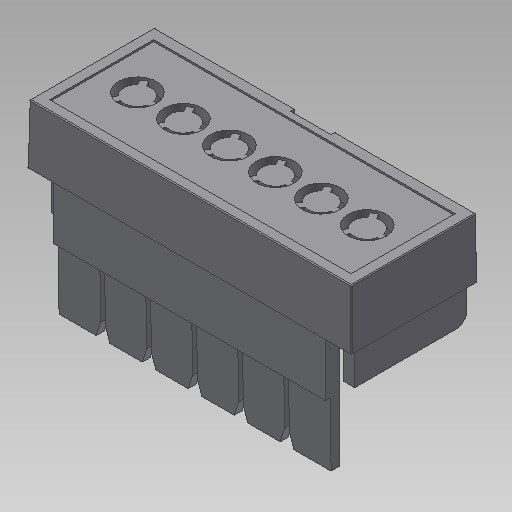
# Autodesk Inventor part: D2MG guard
Saved by Autodesk Inventor 2018 (Build 220112000, 112)
## iProperties
Created: 2015-02-09
Part Number: D2MG guard
Material: Типовые
Document SubType Name: Modeling
Designer: Abbath
Density: 1 g/cm^3
Appearance: По умолчанию
Mass: 2.0666 g
Surface Area: 34.2818 cm^2
Volume: 2.0666 cm^3
Author: Abbath
Autodesk Inventor part; units mm, degrees
ref_plane "YZ Plane" through (0, 0, 0) normal (1, 0, 0) x (0, 1, 0)
ref_plane "XZ Plane" through (0, 0, 0) normal (0, 1, 0) x (-1, 0, 0)
sketch "Эскиз1" plane through (0, 0, 0) normal (0, 0, 1) x (1, 0, 0)
  line L0 (-17.9, 6.95) -> (17.9, 6.95)
  line L1 (17.9, 6.95) -> (17.9, -6.95)
  line L2 (17.9, -6.95) -> (-17.9, -6.95)
  line L3 (-17.9, -6.95) -> (-17.9, 6.95)
  point P0 (0, 0)
  point P1 (17.9, 0)
  point P2 (0, 6.95)
  dimension "d0" = 13.9
  dimension "d1" = 35.8
  constraints: 8 end point, 2 midpoint, 2 parallel, 1 horizontal, 1 horizontal alignment, 1 perpendicular, 1 vertical alignment
  measures "d0" distance between parallel lines of L2 L0
  measures "d1" distance between parallel lines of L1 L3
ref_plane "РабПлоскость1" through (0, 0, 6.5) normal (0, 0, 1) x (1, 0, 0)
sketch "Эскиз2" plane through (0, 0, 6.5) normal (0, 0, 1) x (1, 0, 0)
  line L0 (-17.785, 6.85) -> (17.785, 6.85)
  line L1 (17.785, 6.85) -> (17.785, -6.95)
  line L2 (17.785, -6.95) -> (-17.785, -6.95)
  line L3 (-17.785, -6.95) -> (-17.785, 6.85)
  line L4 (17.9, -6.95) -> (-17.9, -6.95) projected
  point P0 (0, 0)
  point P1 (0, 6.85)
  point P2 (0, -6.95)
  dimension "d3" = 13.8
  dimension "d4" = 35.57
  constraints: 8 end point, 2 midpoint, 2 parallel, 1 collinear, 1 horizontal, 1 perpendicular, 1 vertical alignment
  measures "d3" distance between parallel lines of L2 L0
  measures "d4" distance between parallel lines of L1 L3
loft "Лофт1" add profiles "Эскиз1", "Эскиз2"
sketch "Эскиз3" plane through (-17.9, -6.95, 0) normal (0, -1, 0) x (1, 0, 0)
  line L0 (15.65, 7.5) -> (20.15, 7.5)
  line L1 (20.15, 7.5) -> (20.15, 1)
  line L2 (20.15, 1) -> (15.65, 1)
  line L3 (15.65, 1) -> (15.65, 7.5)
  line L4 (35.8, 0) -> (0, 0) projected
  line L5 (35.685, 6.5) -> (0.115, 6.5) construction
  point P0 (17.9, 0)
  point P1 (17.9, 1)
  point P2 (17.9, 0)
  dimension "d9" = 1
  dimension "d10" = 5.5
  dimension "d11" = 4.5
  constraints: 8 end point, 2 midpoint, 2 parallel, 1 horizontal, 1 perpendicular, 1 vertical alignment
  measures "d9" distance between parallel lines of L5 L0
  measures "d10" distance between parallel lines of L2 L5
  measures "d11" distance between parallel lines of L1 L3
extrude "Выдавливание1" cut sketch "Эскиз3" against normal blind 0.5
sketch "Эскиз4" plane through (-17.785, 6.85, 6.5) normal (0, 0, 1) x (1, 0, 0)
  line L0 (1.135, -1.1) -> (34.435, -1.1)
  line L1 (34.435, -1.1) -> (34.435, -12.6)
  line L2 (34.435, -12.6) -> (1.135, -12.6)
  line L3 (1.135, -12.6) -> (1.135, -1.1)
  point P0 (17.785, -6.85)
  point P1 (34.435, -6.85)
  point P2 (17.785, -1.1)
  dimension "d14" = 11.5
  dimension "d15" = 33.3
  constraints: 8 end point, 2 midpoint, 2 parallel, 1 horizontal, 1 horizontal alignment, 1 perpendicular, 1 vertical alignment
  measures "d14" distance between parallel lines of L2 L0
  measures "d15" distance between parallel lines of L1 L3
extrude "Выдавливание2" cut sketch "Эскиз4" against normal blind 0.2
sketch "Эскиз5" plane through (-17.785, 6.85, 6.3) normal (0, 0, 1) x (1, 0, 0)
  circle A0 centre (5.085, -6.85) radius 2.1
  circle A1 centre (10.165, -6.85) radius 2.1
  circle A2 centre (15.245, -6.85) radius 2.1
  circle A3 centre (20.325, -6.85) radius 2.1
  circle A4 centre (25.405, -6.85) radius 2.1
  circle A5 centre (30.485, -6.85) radius 2.1
  point P0 (17.785, -6.85)
  dimension "d18" = 4.2
  dimension "d19" = 5.08
  dimension "d20" = 2.54
  dimension "d21" = 5.08
  dimension "d22" = 5.08
  dimension "d23" = 5.08
  dimension "d24" = 5.08
  constraints: 6 centre point, 6 horizontal alignment, 5 equal radius
  measures "d18" diameter of A3
  measures "d19" distance of A4.centre A3.centre
  measures "d20" distance of point (17.785, -6.85) A3.centre
  measures "d21" distance of A5.centre A4.centre
  measures "d22" distance of A2.centre A3.centre
  measures "d23" distance of A1.centre A2.centre
  measures "d24" distance of A0.centre A1.centre
extrude "Выдавливание3" cut sketch "Эскиз5" against normal blind 0.3
sketch "Эскиз6" plane through (-12.7, 0, 6) normal (0, 0, 1) x (1, 0, 0)
  circle A0 centre (25.4, 0) radius 2.1 construction
  circle A1 centre (20.32, 0) radius 2.1 construction
  circle A2 centre (15.24, 0) radius 2.1 construction
  circle A3 centre (10.16, 0) radius 2.1 construction
  circle A4 centre (5.08, 0) radius 2.1 construction
  circle A5 centre (0, 0) radius 2.1 construction
  line L0 (25.4, 0) -> (23.3, 0) construction
  line L1 (25.4, 0) -> (26.45, 1.8187) construction
  line L2 (25.4, 0) -> (26.45, -1.8187) construction
  line L3 (20.32, 0) -> (18.22, 0) construction
  line L4 (20.32, 0) -> (21.37, 1.8187) construction
  line L5 (20.32, 0) -> (21.37, -1.8187) construction
  line L6 (15.24, 0) -> (13.14, 0) construction
  line L7 (15.24, 0) -> (16.29, 1.8187) construction
  line L8 (15.24, 0) -> (16.29, -1.8187) construction
  line L9 (10.16, 0) -> (8.06, 0) construction
  line L10 (10.16, 0) -> (11.21, 1.8187) construction
  line L11 (10.16, 0) -> (11.21, -1.8187) construction
  line L12 (5.08, 0) -> (2.98, 0) construction
  line L13 (5.08, 0) -> (6.13, 1.8187) construction
  line L14 (5.08, 0) -> (6.13, -1.8187) construction
  line L15 (0, 0) -> (-2.1, 0) construction
  line L16 (0, 0) -> (1.05, 1.8187) construction
  line L17 (0, 0) -> (1.05, -1.8187) construction
  line L18 (25.8262, 1.4382) -> (26.1322, 1.9682)
  line L19 (26.4324, 1.0882) -> (26.7384, 1.6182)
  line L20 (26.4324, -1.0882) -> (26.7384, -1.6182)
  line L21 (25.8262, -1.4382) -> (26.1322, -1.9682)
  line L22 (23.9414, 0.35) -> (23.3294, 0.35)
  line L23 (23.9414, -0.35) -> (23.3294, -0.35)
  line L24 (20.7462, 1.4382) -> (21.0522, 1.9682)
  line L25 (21.3524, 1.0882) -> (21.6584, 1.6182)
  line L26 (21.3524, -1.0882) -> (21.6584, -1.6182)
  line L27 (20.7462, -1.4382) -> (21.0522, -1.9682)
  line L28 (18.8614, 0.35) -> (18.2494, 0.35)
  line L29 (18.8614, -0.35) -> (18.2494, -0.35)
  line L30 (15.6662, 1.4382) -> (15.9722, 1.9682)
  line L31 (16.2724, 1.0882) -> (16.5784, 1.6182)
  line L32 (16.2724, -1.0882) -> (16.5784, -1.6182)
  line L33 (15.6662, -1.4382) -> (15.9722, -1.9682)
  line L34 (13.7814, 0.35) -> (13.1694, 0.35)
  line L35 (13.7814, -0.35) -> (13.1694, -0.35)
  line L36 (10.5862, 1.4382) -> (10.8922, 1.9682)
  line L37 (11.1924, 1.0882) -> (11.4984, 1.6182)
  line L38 (11.1924, -1.0882) -> (11.4984, -1.6182)
  line L39 (10.5862, -1.4382) -> (10.8922, -1.9682)
  line L40 (8.7014, 0.35) -> (8.0894, 0.35)
  line L41 (8.7014, -0.35) -> (8.0894, -0.35)
  line L42 (5.5062, 1.4382) -> (5.8122, 1.9682)
  line L43 (6.1124, 1.0882) -> (6.4184, 1.6182)
  line L44 (6.1124, -1.0882) -> (6.4184, -1.6182)
  line L45 (5.5062, -1.4382) -> (5.8122, -1.9682)
  line L46 (3.6214, 0.35) -> (3.0094, 0.35)
  line L47 (3.6214, -0.35) -> (3.0094, -0.35)
  line L48 (0.4262, 1.4382) -> (0.7322, 1.9682)
  line L49 (1.0324, 1.0882) -> (1.3384, 1.6182)
  line L50 (1.0324, -1.0882) -> (1.3384, -1.6182)
  line L51 (0.4262, -1.4382) -> (0.7322, -1.9682)
  line L52 (-1.4586, 0.35) -> (-2.0706, 0.35)
  line L53 (-1.4586, -0.35) -> (-2.0706, -0.35)
  arc A6 (1.0324, -1.0882) -> (1.0324, 1.0882) centre (0, 0) ccw
  arc A7 (1.3384, -1.6182) -> (1.3384, 1.6182) centre (0, 0) ccw
  arc A8 (0.7322, 1.9682) -> (-2.0706, 0.35) centre (0, 0) ccw
  arc A9 (-2.0706, -0.35) -> (0.7322, -1.9682) centre (0, 0) ccw
  arc A10 (0.4262, 1.4382) -> (-1.4586, 0.35) centre (0, 0) ccw
  arc A11 (-1.4586, -0.35) -> (0.4262, -1.4382) centre (0, 0) ccw
  arc A12 (26.4324, -1.0882) -> (26.4324, 1.0882) centre (25.4, 0) ccw
  arc A13 (26.7384, -1.6182) -> (26.7384, 1.6182) centre (25.4, 0) ccw
  arc A14 (25.8262, 1.4382) -> (23.9414, 0.35) centre (25.4, 0) ccw
  arc A15 (23.9414, -0.35) -> (25.8262, -1.4382) centre (25.4, 0) ccw
  arc A16 (26.1322, 1.9682) -> (23.3294, 0.35) centre (25.4, 0) ccw
  arc A17 (23.3294, -0.35) -> (26.1322, -1.9682) centre (25.4, 0) ccw
  arc A18 (21.0522, 1.9682) -> (18.2494, 0.35) centre (20.32, 0) ccw
  arc A19 (20.7462, 1.4382) -> (18.8614, 0.35) centre (20.32, 0) ccw
  arc A20 (18.8614, -0.35) -> (20.7462, -1.4382) centre (20.32, 0) ccw
  arc A21 (21.3524, -1.0882) -> (21.3524, 1.0882) centre (20.32, 0) ccw
  arc A22 (18.2494, -0.35) -> (21.0522, -1.9682) centre (20.32, 0) ccw
  arc A23 (21.6584, -1.6182) -> (21.6584, 1.6182) centre (20.32, 0) ccw
  arc A24 (13.1694, -0.35) -> (15.9722, -1.9682) centre (15.24, 0) ccw
  arc A25 (13.7814, -0.35) -> (15.6662, -1.4382) centre (15.24, 0) ccw
  arc A26 (16.2724, -1.0882) -> (16.2724, 1.0882) centre (15.24, 0) ccw
  arc A27 (15.6662, 1.4382) -> (13.7814, 0.35) centre (15.24, 0) ccw
  arc A28 (16.5784, -1.6182) -> (16.5784, 1.6182) centre (15.24, 0) ccw
  arc A29 (15.9722, 1.9682) -> (13.1694, 0.35) centre (15.24, 0) ccw
  arc A30 (11.1924, -1.0882) -> (11.1924, 1.0882) centre (10.16, 0) ccw
  arc A31 (11.4984, -1.6182) -> (11.4984, 1.6182) centre (10.16, 0) ccw
  arc A32 (10.5862, 1.4382) -> (8.7014, 0.35) centre (10.16, 0) ccw
  arc A33 (8.7014, -0.35) -> (10.5862, -1.4382) centre (10.16, 0) ccw
  arc A34 (10.8922, 1.9682) -> (8.0894, 0.35) centre (10.16, 0) ccw
  arc A35 (8.0894, -0.35) -> (10.8922, -1.9682) centre (10.16, 0) ccw
  arc A36 (6.1124, -1.0882) -> (6.1124, 1.0882) centre (5.08, 0) ccw
  arc A37 (6.4184, -1.6182) -> (6.4184, 1.6182) centre (5.08, 0) ccw
  arc A38 (5.5062, 1.4382) -> (3.6214, 0.35) centre (5.08, 0) ccw
  arc A39 (3.6214, -0.35) -> (5.5062, -1.4382) centre (5.08, 0) ccw
  arc A40 (5.8122, 1.9682) -> (3.0094, 0.35) centre (5.08, 0) ccw
  arc A41 (3.0094, -0.35) -> (5.8122, -1.9682) centre (5.08, 0) ccw
  point P0 (12.7, 0)
  dimension "d27" = 120
  dimension "d28" = 120
  dimension "d29" = 0.7
  dimension "d30" = 0.35
  dimension "d31" = 0.6
  dimension "d32" = 0.35
  dimension "d33" = 0.7
  dimension "d34" = 0.7
  dimension "d36" = 0.35
  constraints: 108 end point, 90 point on circle, 46 parallel, 36 centre point, 34 equal radius, 30 equal length, 13 horizontal, 12 coincident, 5 point on line, 1 concentric
  measures "d27" angle of L16 L15
  measures "d28" angle of L17 L15
  measures "d29" distance between parallel lines of L49 L48
  measures "d30" distance between parallel lines of L16 L48
  measures "d31" radial gap between concentric circles of A6 A7
  measures "d32" distance between parallel lines of L17 L50
  measures "d33" distance between parallel lines of L51 L50
  measures "d34" distance between parallel lines of L53 L52
  measures "d36" distance between parallel lines of L15 L52
extrude "Выдавливание4" cut sketch "Эскиз6" against normal through all
sketch "Эскиз7" plane through (17.9, 6.95, 0) normal (0, 0, -1) x (-1, 0, 0)
  line L0 (2.875, 0) -> (32.925, 0)
  line L1 (32.925, 0) -> (32.925, -1.5)
  line L2 (32.925, -1.5) -> (2.875, -1.5)
  line L3 (2.875, -1.5) -> (2.875, 0)
  line L4 (35.8, 0) -> (0, 0) construction
  point P0 (17.9, -6.95)
  point P1 (17.9, -1.5)
  dimension "d39" = 1.5
  dimension "d40" = 30.05
  constraints: 8 end point, 2 parallel, 1 collinear, 1 horizontal, 1 midpoint, 1 perpendicular, 1 vertical alignment
  measures "d39" distance between parallel lines of L2 L4
  measures "d40" distance between parallel lines of L1 L3
extrude "Выдавливание5" add sketch "Эскиз7" along normal blind 12.9
sketch "Эскиз8" plane through (0, 0, 0) normal (1, 0, 0) x (0, 1, 0)
  line L0 (6.33, -12.9) -> (6.42, -5.85)
  line L1 (6.42, -5.85) -> (6.95, -5.85)
  line L2 (5.45, 0) -> (5.45, -12.9) projected
  line L3 (6.95, -5.85) -> (6.95, -12.9)
  line L4 (6.95, -12.9) -> (6.33, -12.9)
  line L5 (6.95, -12.9) -> (5.45, -12.9) construction
  line L6 (6.95, 0) -> (6.95, -12.9) construction
  point P0 (0, 0)
  dimension "d43" = 0.53
  dimension "d44" = 0.88
  dimension "d45" = 7.05
  constraints: 8 end point, 3 perpendicular, 2 collinear
  measures "d43" distance from line of L0.end L3
  measures "d44" distance from line of L0.start L2
  measures "d45" distance from line of L1 L0.start
extrude "Выдавливание6" cut sketch "Эскиз8" along normal through all both and the other way through all
sketch "Эскиз9" plane through (-15.025, 5.45, 0) normal (0, -1, 0) x (1, 0, 0)
  line L0 (30.05, -5.85) -> (0, -5.85) construction
  line L1 (4.865, -4.0724) -> (4.865, -15.392) construction
  line L2 (9.945, -3.6307) -> (9.945, -16.2754) construction
  line L3 (15.025, -4.0724) -> (15.025, -16.2754) construction
  line L4 (20.105, -4.0724) -> (20.105, -15.392) construction
  line L5 (25.185, -3.6307) -> (25.185, -16.2754) construction
  line L6 (30.05, 0) -> (30.05, -12.9) construction
  line L7 (0, 0) -> (0, -12.9) construction
  line L8 (4.115, -12.9) -> (4.6, -11.4)
  line L9 (4.6, -11.4) -> (4.6, -5.85)
  line L10 (31.675, 6.3) -> (31.675, 6.5) construction
  line L11 (31.675, 6.5) -> (32.81, 6.5) construction
  line L12 (32.81, 6.5) -> (32.925, 0) construction
  line L13 (32.925, 0) -> (30.05, 0) construction
  line L14 (30.05, 0) -> (30.05, -12.9) construction
  line L15 (30.05, -12.9) -> (0, -12.9) construction
  line L16 (0, -12.9) -> (0, 0) construction
  line L17 (0, 0) -> (-2.875, 0) construction
  line L18 (-2.875, 0) -> (-2.76, 6.5) construction
  line L19 (-2.76, 6.5) -> (-1.625, 6.5) construction
  line L20 (-1.625, 6.5) -> (-1.625, 6.3) construction
  line L21 (-1.625, 6.3) -> (31.675, 6.3) construction
  line L22 (30.05, 0) -> (0, 0) construction
  line L23 (4.6, -5.85) -> (5.13, -5.85)
  line L24 (5.13, -5.85) -> (5.13, -11.4)
  line L25 (5.615, -12.9) -> (9.195, -12.9)
  line L26 (5.13, -11.4) -> (5.615, -12.9)
  line L27 (9.195, -12.9) -> (9.68, -11.4)
  line L28 (9.68, -11.4) -> (9.68, -5.85)
  line L29 (9.68, -5.85) -> (10.21, -5.85)
  line L30 (10.21, -5.85) -> (10.21, -11.4)
  line L31 (10.21, -11.4) -> (10.695, -12.9)
  line L32 (10.695, -12.9) -> (14.275, -12.9)
  line L33 (14.275, -12.9) -> (14.76, -11.4)
  line L34 (14.76, -11.4) -> (14.76, -5.85)
  line L35 (14.76, -5.85) -> (15.29, -5.85)
  line L36 (15.29, -5.85) -> (15.29, -11.4)
  line L37 (15.29, -11.4) -> (15.775, -12.9)
  line L38 (15.775, -12.9) -> (19.355, -12.9)
  line L39 (19.355, -12.9) -> (19.84, -11.4)
  line L40 (19.84, -11.4) -> (19.84, -5.85)
  line L41 (19.84, -5.85) -> (20.37, -5.85)
  line L42 (20.37, -5.85) -> (20.37, -11.4)
  line L43 (20.37, -11.4) -> (20.855, -12.9)
  line L44 (20.855, -12.9) -> (24.435, -12.9)
  line L45 (24.435, -12.9) -> (24.92, -11.4)
  line L46 (24.92, -11.4) -> (24.92, -5.85)
  line L47 (24.92, -5.85) -> (25.45, -5.85)
  line L48 (25.45, -5.85) -> (25.45, -11.4)
  line L49 (25.45, -11.4) -> (25.935, -12.9)
  line L50 (25.935, -12.9) -> (25.935, -13.9)
  line L51 (25.935, -13.9) -> (4.115, -13.9)
  line L52 (4.115, -13.9) -> (4.115, -12.9)
  point P0 (15.025, 0)
  point P1 (9.945, -5.85)
  point P2 (15.025, -5.85)
  point P3 (20.105, -5.85)
  point P4 (25.185, -5.85)
  dimension "d48" = 5.08
  dimension "d49" = 5.08
  dimension "d50" = 5.08
  dimension "d51" = 5.08
  dimension "d52" = 4.865
  dimension "d53" = 4.865
  dimension "d54" = 0.53
  dimension "d55" = 0.265
  dimension "d57" = 1
  dimension "d58" = 1.5
  dimension "d59" = 1.5
  constraints: 74 end point, 13 perpendicular, 10 equal length, 9 horizontal alignment, 9 vertical, 8 collinear, 8 point on line, 4 midpoint, 4 parallel, 3 horizontal
  measures "d48" distance between parallel lines of L5 L4
  measures "d49" distance between parallel lines of L3 L4
  measures "d50" distance between parallel lines of L2 L3
  measures "d51" distance between parallel lines of L1 L2
  measures "d52" distance between parallel lines of L6 L5
  measures "d53" distance between parallel lines of L7 L1
  measures "d54" distance between parallel lines of L24 L9
  measures "d55" distance between parallel lines of L1 L9
  measures "d57" distance between parallel lines of L51 L15
  measures "d58" distance from line of L8.end L15
  measures "d59" distance of L25.start L8.start
extrude "Выдавливание7" cut sketch "Эскиз9" against normal through all
sketch "Эскиз10" plane through (17.9, -6.95, 0) normal (0, 0, -1) x (-1, 0, 0)
  line L0 (33.45, 12.4) -> (2.35, 12.4)
  line L1 (2.35, 12.4) -> (2.35, 1.5)
  line L2 (2.35, 1.5) -> (33.45, 1.5)
  line L3 (33.45, 1.5) -> (33.45, 12.4)
  line L4 (35.8, 0) -> (35.8, 13.9) projected
  line L5 (0, 0) -> (35.8, 0) projected
  line L6 (0, 13.9) -> (0, 0) projected
  line L7 (28.81, 12.4) -> (32.925, 12.4) projected
  point P0 (17.9, 6.95)
  point P1 (17.9, 1.5)
  dimension "d63" = 1.5
  dimension "d70" = 31.1
  constraints: 8 end point, 2 parallel, 1 collinear, 1 horizontal, 1 midpoint, 1 perpendicular, 1 vertical alignment
  measures "d63" distance between parallel lines of L5 L2
  measures "d70" distance between parallel lines of L1 L3
extrude "Выдавливание8" cut sketch "Эскиз10" against normal blind 5
sketch "Эскиз11" plane through (17.9, -6.95, 0) normal (0, 0, -1) x (-1, 0, 0)
  line L0 (32.9, 0) -> (2.9, 0)
  line L1 (2.9, 0) -> (2.9, 1.5)
  line L2 (2.9, 1.5) -> (32.9, 1.5)
  line L3 (32.9, 1.5) -> (32.9, 0)
  line L4 (33.45, 1.5) -> (2.35, 1.5) projected
  line L5 (0, 0) -> (35.8, 0) projected
  point P0 (17.9, 6.95)
  point P1 (17.9, 0)
  dimension "d67" = 30
  constraints: 8 end point, 2 collinear, 2 parallel, 1 horizontal, 1 midpoint, 1 perpendicular, 1 vertical alignment
  measures "d67" distance between parallel lines of L1 L3
extrude "Выдавливание9" add sketch "Эскиз11" along normal blind 3.5
sketch "Эскиз12" plane through (-15.55, -5.45, 5) normal (0, 1, 0) x (1, 0, 0)
  line L0 (31.1, 0) -> (0, 0) construction
  line L1 (31.1, 5) -> (31.1, 0) construction
  line L2 (0, 5) -> (0, 0) construction
  line L3 (0.18, 0) -> (1.38, 0)
  line L4 (1.38, 0) -> (2, 8.5)
  line L5 (2, 8.5) -> (29.1, 8.5)
  line L6 (29.1, 8.5) -> (29.72, 0)
  line L7 (29.72, 0) -> (30.92, 0)
  line L8 (31.1, 9.5) -> (0, 9.5)
  line L9 (30.92, 0) -> (31.1, 5)
  line L10 (31.1, 5) -> (31.1, 9.5)
  line L11 (0.18, 0) -> (0, 5)
  line L12 (0, 5) -> (0, 9.5)
  line L13 (30.55, 8.5) -> (0.55, 8.5) projected
  point P0 (15.55, 5)
  dimension "d71" = 0.18
  dimension "d72" = 1.2
  dimension "d73" = 2
  dimension "d74" = 1
  constraints: 21 end point, 3 collinear, 3 equal length, 2 vertical, 1 horizontal
  measures "d71" distance from line of L3.start L12
  measures "d72" distance of L3.end L3.start
  measures "d73" horizontal distance of L4.end L2.start
  measures "d74" distance between parallel lines of L8 L13
extrude "Выдавливание10" cut sketch "Эскиз12" against normal through all
sketch "Эскиз13" plane through (0, 0, 0) normal (1, 0, 0) x (0, 1, 0)
  line L0 (-6.95, 0) -> (-6.95, -2)
  line L1 (-6.95, -2) -> (-7.75, 0)
  line L2 (-7.75, 0) -> (-6.95, 0)
  line L3 (-6.95, -3.5) -> (-6.95, 5) projected
  line L4 (6.95, 0) -> (-6.95, 0) construction
  point P0 (0, 0)
  dimension "d77" = 2
  dimension "d78" = 0.8
  constraints: 6 end point, 2 collinear, 1 perpendicular, 1 vertical
  measures "d77" distance from line of L0.end L2
  measures "d78" distance of L1.end L0.start
extrude "Выдавливание11" add sketch "Эскиз13" along normal mid plane 3
sketch "Эскиз14" plane through (2.25, -6.95, 6.5) normal (0, -1, 0) x (1, 0, 0)
  line L0 (-17.8, -11) -> (-17.8, -6.5)
  line L1 (-17.8, -6.5) -> (-19, -6.5)
  line L2 (-19, -6.5) -> (-19, -11)
  line L3 (-19, -11) -> (-17.8, -11)
  line L4 (13.3, -11) -> (13.3, -6.5)
  line L5 (13.3, -6.5) -> (14.5, -6.5)
  line L6 (14.5, -6.5) -> (14.5, -11)
  line L7 (14.5, -11) -> (13.3, -11)
  line L8 (-4.5, 0) -> (-20.035, 0) construction
  point P0 (-2.25, -6.5)
  dimension "d83" = 1.2
  dimension "d101" = 11
  constraints: 16 end point, 3 collinear, 3 vertical, 2 coincident, 2 parallel, 2 perpendicular
  measures "d83" distance of L0.end L1.end
  measures "d101" distance between parallel lines of L3 L8
extrude "Выдавливание12" add sketch "Эскиз14" against normal blind 12.4
fillet "Сопряжение6" radius 0.1 9 edges at (17.8425, 6.9, 3.25) (-17.8425, 6.9, 3.25) (17.8425, -6.95, 3.25) (-17.8425, -6.95, 3.25) (-17.785, -0.05, 6.5) (-10.0175, -6.95, 6.5) (10.0175, -6.95, 6.5) (17.785, -0.05, 6.5) (0, 6.85, 6.5)
fillet "Сопряжение7" radius 1.2 2 edges at (-16.15, -6.95, -4.5) (16.15, -6.95, -4.5)
equation "\"d20\" = 0.5 * d19"
equation "\"d21\" = d19"
equation "\"d22\" = d19"
equation "\"d23\" = d19"
equation "\"d24\" = d19"
equation "\"d30\" = 0.5 * d29"
equation "\"d32\" = d30"
equation "\"d33\" = d29"
equation "\"d34\" = d29"
equation "\"d36\" = d30"
equation "\"d49\" = d48"
equation "\"d50\" = d49"
equation "\"d51\" = d50"
equation "\"d52\" = d53"
equation "\"d55\" = 0.5 * d54"
equation "\"d63\" = d62"
equation "\"d62\" = 1.5"
